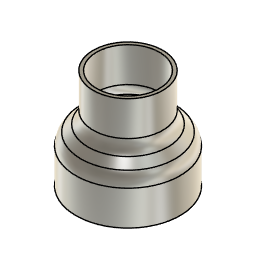
drop_saw_dust_extracion_adapter (Autodesk Fusion 360 design; units mm, degrees)
Autodesk Fusion 360 part; units mm, degrees
sketch "Sketch1" plane through (0, 0, 0) normal (0, 0, 1) x (1, 0, 0)
  circle A0 centre (0, 0) radius 29.25
  circle A1 centre (0, 0) radius 31.25
  dimension "d1" = 58.5
  dimension "d2" = 2
  constraint coincident A0.centre A1.centre
  measures "d1" diameter of A0
ref_plane "WorkPlane1" through (0, 0, 10) normal (0, 0, 1) x (1, 0, 0)
sketch "Sketch2" plane through (0, 0, 10) normal (0, 0, 1) x (1, 0, 0)
  circle A0 centre (0, 0) radius 18.9
  circle A1 centre (0, 0) radius 20.9
  dimension "d4" = 37.8
  dimension "d5" = 2
  constraint coincident A0.centre A1.centre
  measures "d4" diameter of A0
sketch "Sketch3" plane through (0, 0, 0) normal (0, 1, 0) x (1, 0, 0)
  line L0 (-29.25, 0) -> (29.25, 0)
  line L1 (-31.25, 0) -> (31.25, 0)
  line L2 (-18.9, -10) -> (18.9, -10)
  line L3 (-20.9, -10) -> (20.9, -10)
  line L4 (-31.25, 0) -> (-20.9, -10)
  line L5 (-18.9, -10) -> (-29.25, 0)
  line L6 (0, 0) -> (0, -30) construction
  constraint coincident L1.start L4.start
  constraint coincident L3.start L4.end
  constraint coincident L2.start L5.start
  constraint coincident L0.start L5.end
  constraint coincident L6.start origin
  constraint perpendicular L0 L6
revolve "Revolve1" add sketch "Sketch3" angle 360 about axis through (0, 0, 0) along (0, 0, 1)
extrude "Extrude1" add sketch "Sketch2" along normal blind 25
extrude "Extrude2" add sketch "Sketch1" against normal blind 25
fillet "Fillet1" radius 10 1 edges at (-27.2706, 10.5773, 0)
fillet "Fillet2" radius 10 2 edges at (-17.621, 6.8345, 10) (-19.4856, 7.5578, 10)
fillet "Fillet3" radius 10 1 edges at (-29.1352, 11.3005, 0)
